Autodesk Fusion 360 part; units mm, degrees
note: some values were not read from the file. Set by a fixed rule: which face or edge a step refers to.
(part 20 of 20)
  spline S58 degree 5 poles (-8.3931, 13.6219) (-8.3929, 13.6198) (-8.3924, 13.6155) (-8.3916, 13.6092) (-8.3906, 13.6008) (-8.3893, 13.5903) (-8.3879, 13.5798) (-8.3866, 13.5693) (-8.3853, 13.5589) (-8.3839, 13.5485) (-8.3826, 13.5382) (-8.3812, 13.5278) (-8.3798, 13.5175) (-8.3784, 13.5072) (-8.377, 13.497) (-8.3755, 13.4867) (-8.3741, 13.4766) (-8.3726, 13.4664) (-8.3712, 13.4563) (-8.3697, 13.4461) (-8.3682, 13.4361) (-8.3667, 13.426) (-8.3652, 13.416) (-8.3637, 13.406) (-8.3621, 13.396) (-8.3606, 13.3861) (-8.359, 13.3762) (-8.3574, 13.3663) (-8.3558, 13.3565) (-8.3542, 13.3467) (-8.3526, 13.3369) (-8.351, 13.3272) (-8.3494, 13.3174) (-8.3477, 13.3078) (-8.3461, 13.2981) (-8.3444, 13.2885) (-8.3427, 13.2789) (-8.341, 13.2693) (-8.3393, 13.2598) (-8.3376, 13.2503) (-8.3359, 13.2408) (-8.3342, 13.2313) (-8.3324, 13.2219) (-8.3307, 13.2125) (-8.3289, 13.2032) (-8.3271, 13.1939) (-8.3254, 13.1846) (-8.3236, 13.1753) (-8.3218, 13.1661) (-8.3199, 13.1569) (-8.3181, 13.1478) (-8.3163, 13.1386) (-8.3145, 13.1296) (-8.3126, 13.1205) (-8.3107, 13.1115) (-8.3089, 13.1025) (-8.307, 13.0935) (-8.3051, 13.0846) (-8.3032, 13.0757) (-8.3013, 13.0668) (-8.2994, 13.058) (-8.2975, 13.0492) (-8.2956, 13.0404) (-8.2936, 13.0317) (-8.2917, 13.023) (-8.2897, 13.0143) (-8.2878, 13.0057) (-8.2858, 12.9971) (-8.2838, 12.9885) (-8.2818, 12.98) (-8.2799, 12.9715) (-8.2779, 12.963) (-8.2759, 12.9546) (-8.2738, 12.9462) (-8.2718, 12.9379) (-8.2698, 12.9295) (-8.2678, 12.9212) (-8.2657, 12.913) (-8.2637, 12.9048) (-8.2616, 12.8966) (-8.2596, 12.8884) (-8.2575, 12.8803) (-8.2554, 12.8722) (-8.2534, 12.8642) (-8.2513, 12.8562) (-8.2492, 12.8482) (-8.2471, 12.8403) (-8.245, 12.8324) (-8.2429, 12.8245) (-8.2408, 12.8167) (-8.2387, 12.8089) (-8.2366, 12.8011) (-8.2345, 12.7934) (-8.2323, 12.7857) (-8.2302, 12.7781) (-8.2281, 12.7705) (-8.2259, 12.7629) (-8.2238, 12.7554) (-8.2216, 12.7479) (-8.2195, 12.7404) (-8.2173, 12.733) (-8.2152, 12.7256) (-8.213, 12.7183) (-8.2109, 12.711) (-8.2087, 12.7037) (-8.2065, 12.6965) (-8.2044, 12.6893) (-8.2022, 12.6821) (-8.2, 12.675) (-8.1978, 12.6679) (-8.1956, 12.6609) (-8.1935, 12.6539) (-8.1913, 12.6469) (-8.1891, 12.64) (-8.1869, 12.6331) (-8.1847, 12.6263) (-8.1825, 12.6195) (-8.1803, 12.6127) (-8.1782, 12.606) (-8.176, 12.5993) (-8.1738, 12.5926) (-8.1716, 12.586) (-8.1694, 12.5795) (-8.1672, 12.5729) (-8.165, 12.5665) (-8.1628, 12.56) (-8.1606, 12.5536) (-8.1584, 12.5473) (-8.1563, 12.5409) (-8.1541, 12.5347) (-8.1519, 12.5284) (-8.1497, 12.5222) (-8.1475, 12.5161) (-8.1453, 12.51) (-8.1432, 12.5039) (-8.141, 12.4979) (-8.1388, 12.4919) (-8.1366, 12.4859) (-8.1345, 12.48) (-8.1323, 12.4742) (-8.1302, 12.4683) (-8.128, 12.4626) (-8.1258, 12.4568) (-8.1237, 12.4512) (-8.1215, 12.4455) (-8.1194, 12.4399) (-8.1173, 12.4344) (-8.1151, 12.4289) (-8.113, 12.4234) (-8.1109, 12.418) (-8.1088, 12.4126) (-8.1067, 12.4073) (-8.1046, 12.402) (-8.1025, 12.3967) (-8.1004, 12.3915) (-8.0983, 12.3864) (-8.0962, 12.3813) (-8.0941, 12.3762) (-8.0921, 12.3712) (-8.09, 12.3662) (-8.088, 12.3613) (-8.0859, 12.3564) (-8.0839, 12.3516) (-8.0819, 12.3468) (-8.0799, 12.3421) (-8.0779, 12.3374) (-8.0759, 12.3327) (-8.0739, 12.3281) (-8.0719, 12.3236) (-8.0699, 12.3191) (-8.068, 12.3146) (-8.066, 12.3102) (-8.0641, 12.3059) (-8.0622, 12.3016) (-8.0603, 12.2973) (-8.0584, 12.2931) (-8.0565, 12.289) (-8.0546, 12.2848) (-8.0527, 12.2808) (-8.0509, 12.2768) (-8.0491, 12.2728) (-8.0472, 12.2689) (-8.0454, 12.265) (-8.0436, 12.2612) (-8.0419, 12.2575) (-8.0401, 12.2538) (-8.0383, 12.2501) (-8.0366, 12.2465) (-8.0349, 12.243) (-8.0332, 12.2395) (-8.0315, 12.236) (-8.0298, 12.2326) (-8.0282, 12.2293) (-8.0265, 12.226) (-8.0249, 12.2228) (-8.0233, 12.2196) (-8.0218, 12.2164) (-8.0202, 12.2134) (-8.0187, 12.2104) (-8.0171, 12.2074) (-8.0156, 12.2045) (-8.0142, 12.2016) (-8.0127, 12.1988) (-8.0113, 12.1961) (-8.0098, 12.1934) (-8.0084, 12.1908) (-8.0071, 12.1882) (-8.0057, 12.1857) (-8.0044, 12.1832) (-8.0031, 12.1808) (-8.0018, 12.1785) (-8.0006, 12.1762) (-7.9994, 12.1739) (-7.9982, 12.1718) (-7.997, 12.1696) (-7.9958, 12.1676) (-7.9947, 12.1656) (-7.9936, 12.1637) (-7.9926, 12.1618) (-7.9915, 12.16) (-7.9905, 12.1582) (-7.9896, 12.1565) (-7.9886, 12.1549) (-7.9877, 12.1533) (-7.9868, 12.1518) (-7.986, 12.1504) (-7.9852, 12.149) (-7.9844, 12.1477) (-7.9836, 12.1464) (-7.9829, 12.1452) (-7.9823, 12.1441) (-7.9816, 12.1431) (-7.981, 12.1421) (-7.9804, 12.1411) (-7.9799, 12.1403) (-7.9794, 12.1395) (-7.979, 12.1388) (-7.9786, 12.1381) (-7.9782, 12.1375) (-7.9779, 12.137) (-7.9776, 12.1365) (-7.9774, 12.1362) (-7.9772, 12.136) (-7.9772, 12.1359) (-7.9771, 12.1359) knots -1 -1 -1 -1 -1 -1 -0.99583333 -0.99166667 -0.9875 -0.98333333 -0.97916667 -0.975 -0.97083333 -0.96666667 -0.9625 -0.95833333 -0.95416667 -0.95 -0.94583333 -0.94166667 -0.9375 -0.93333333 -0.92916667 -0.925 -0.92083333 -0.91666667 -0.9125 -0.90833333 -0.90416667 -0.9 -0.89583333 -0.89166667 -0.8875 -0.88333333 -0.87916667 -0.875 -0.87083333 -0.86666667 -0.8625 -0.85833333 -0.85416667 -0.85 -0.84583333 -0.84166667 -0.8375 -0.83333333 -0.82916667 -0.825 -0.82083333 -0.81666667 -0.8125 -0.80833333 -0.80416667 -0.8 -0.79583333 -0.79166667 -0.7875 -0.78333333 -0.77916667 -0.775 -0.77083333 -0.76666667 -0.7625 -0.75833333 -0.75416667 -0.75 -0.74583333 -0.74166667 -0.7375 -0.73333333 -0.72916667 -0.725 -0.72083333 -0.71666667 -0.7125 -0.70833333 -0.70416667 -0.7 -0.69583333 -0.69166667 -0.6875 -0.68333333 -0.67916667 -0.675 -0.67083333 -0.66666667 -0.6625 -0.65833333 -0.65416667 -0.65 -0.64583333 -0.64166667 -0.6375 -0.63333333 -0.62916667 -0.625 -0.62083333 -0.61666667 -0.6125 -0.60833333 -0.60416667 -0.6 -0.59583333 -0.59166667 -0.5875 -0.58333333 -0.57916667 -0.575 -0.57083333 -0.56666667 -0.5625 -0.55833333 -0.55416667 -0.55 -0.54583333 -0.54166667 -0.5375 -0.53333333 -0.52916667 -0.525 -0.52083333 -0.51666667 -0.5125 -0.50833333 -0.50416667 -0.5 -0.49583333 -0.49166667 -0.4875 -0.48333333 -0.47916667 -0.475 -0.47083333 -0.46666667 -0.4625 -0.45833333 -0.45416667 -0.45 -0.44583333 -0.44166667 -0.4375 -0.43333333 -0.42916667 -0.425 -0.42083333 -0.41666667 -0.4125 -0.40833333 -0.40416667 -0.4 -0.39583333 -0.39166667 -0.3875 -0.38333333 -0.37916667 -0.375 -0.37083333 -0.36666667 -0.3625 -0.35833333 -0.35416667 -0.35 -0.34583333 -0.34166667 -0.3375 -0.33333333 -0.32916667 -0.325 -0.32083333 -0.31666667 -0.3125 -0.30833333 -0.30416667 -0.3 -0.29583333 -0.29166667 -0.2875 -0.28333333 -0.27916667 -0.275 -0.27083333 -0.26666667 -0.2625 -0.25833333 -0.25416667 -0.25 -0.24583333 -0.24166667 -0.2375 -0.23333333 -0.22916667 -0.225 -0.22083333 -0.21666667 -0.2125 -0.20833333 -0.20416667 -0.2 -0.19583333 -0.19166667 -0.1875 -0.18333333 -0.17916667 -0.175 -0.17083333 -0.16666667 -0.1625 -0.15833333 -0.15416667 -0.15 -0.14583333 -0.14166667 -0.1375 -0.13333333 -0.12916667 -0.125 -0.12083333 -0.11666667 -0.1125 -0.10833333 -0.10416667 -0.1 -0.09583333 -0.09166667 -0.0875 -0.08333333 -0.07916667 -0.075 -0.07083333 -0.06666667 -0.0625 -0.05833333 -0.05416667 -0.05 -0.04583333 -0.04166667 -0.0375 -0.03333333 -0.02916667 -0.025 -0.02083333 -0.01666667 -0.0125 -0.00833333 -0.00416667 0 0 0 0 0 0
  line L116 (-7.9771, 12.1359) -> (-7.9768, 12.1353)
  line L117 (-7.9768, 12.1353) -> (-7.5526, 11.49)
  arc A58 (-7.5526, 11.49) -> (-8.5938, 10.7336) centre (0, 0) ccw
  line L118 (-8.5938, 10.7336) -> (-9.0764, 11.3364)
  line L119 (-9.0764, 11.3364) -> (-9.0768, 11.3369)
  spline S59 degree 5 poles (-9.0768, 11.3369) (-9.0769, 11.3369) (-9.0769, 11.337) (-9.0771, 11.3372) (-9.0773, 11.3375) (-9.0777, 11.3379) (-9.0781, 11.3384) (-9.0785, 11.3389) (-9.079, 11.3395) (-9.0796, 11.3402) (-9.0802, 11.3409) (-9.0808, 11.3417) (-9.0815, 11.3425) (-9.0823, 11.3434) (-9.0831, 11.3443) (-9.084, 11.3453) (-9.0849, 11.3464) (-9.0858, 11.3475) (-9.0868, 11.3486) (-9.0879, 11.3498) (-9.089, 11.3511) (-9.0902, 11.3524) (-9.0914, 11.3537) (-9.0926, 11.3551) (-9.0939, 11.3566) (-9.0953, 11.3581) (-9.0967, 11.3596) (-9.0982, 11.3612) (-9.0997, 11.3628) (-9.1012, 11.3645) (-9.1028, 11.3662) (-9.1045, 11.368) (-9.1062, 11.3698) (-9.1079, 11.3717) (-9.1097, 11.3735) (-9.1115, 11.3755) (-9.1134, 11.3775) (-9.1153, 11.3795) (-9.1173, 11.3815) (-9.1194, 11.3836) (-9.1214, 11.3858) (-9.1235, 11.388) (-9.1257, 11.3902) (-9.1279, 11.3924) (-9.1302, 11.3947) (-9.1325, 11.397) (-9.1348, 11.3994) (-9.1372, 11.4018) (-9.1397, 11.4042) (-9.1422, 11.4067) (-9.1447, 11.4092) (-9.1473, 11.4117) (-9.1499, 11.4143) (-9.1526, 11.4169) (-9.1553, 11.4195) (-9.158, 11.4222) (-9.1608, 11.4249) (-9.1637, 11.4276) (-9.1666, 11.4304) (-9.1695, 11.4332) (-9.1725, 11.436) (-9.1755, 11.4389) (-9.1786, 11.4418) (-9.1817, 11.4447) (-9.1848, 11.4476) (-9.188, 11.4506) (-9.1913, 11.4536) (-9.1946, 11.4566) (-9.1979, 11.4597) (-9.2013, 11.4627) (-9.2047, 11.4658) (-9.2081, 11.469) (-9.2116, 11.4721) (-9.2152, 11.4753) (-9.2188, 11.4785) (-9.2224, 11.4818) (-9.2261, 11.485) (-9.2298, 11.4883) (-9.2335, 11.4916) (-9.2373, 11.495) (-9.2412, 11.4983) (-9.2451, 11.5017) (-9.249, 11.5051) (-9.253, 11.5085) (-9.257, 11.512) (-9.261, 11.5154) (-9.2651, 11.5189) (-9.2692, 11.5224) (-9.2734, 11.526) (-9.2776, 11.5295) (-9.2819, 11.5331) (-9.2862, 11.5367) (-9.2905, 11.5403) (-9.2949, 11.544) (-9.2993, 11.5476) (-9.3038, 11.5513) (-9.3083, 11.555) (-9.3128, 11.5587) (-9.3174, 11.5624) (-9.322, 11.5662) (-9.3267, 11.5699) (-9.3314, 11.5737) (-9.3361, 11.5775) (-9.3409, 11.5813) (-9.3457, 11.5852) (-9.3506, 11.589) (-9.3555, 11.5929) (-9.3605, 11.5968) (-9.3654, 11.6007) (-9.3705, 11.6046) (-9.3755, 11.6085) (-9.3806, 11.6125) (-9.3858, 11.6164) (-9.3909, 11.6204) (-9.3962, 11.6244) (-9.4014, 11.6284) (-9.4067, 11.6324) (-9.412, 11.6365) (-9.4174, 11.6405) (-9.4228, 11.6446) (-9.4283, 11.6486) (-9.4338, 11.6527) (-9.4393, 11.6568) (-9.4449, 11.6609) (-9.4505, 11.6651) (-9.4561, 11.6692) (-9.4618, 11.6733) (-9.4675, 11.6775) (-9.4733, 11.6817) (-9.4791, 11.6859) (-9.4849, 11.6901) (-9.4908, 11.6943) (-9.4967, 11.6985) (-9.5026, 11.7027) (-9.5086, 11.707) (-9.5146, 11.7112) (-9.5207, 11.7155) (-9.5268, 11.7197) (-9.5329, 11.724) (-9.5391, 11.7283) (-9.5453, 11.7326) (-9.5516, 11.7369) (-9.5578, 11.7412) (-9.5642, 11.7455) (-9.5705, 11.7499) (-9.5769, 11.7542) (-9.5833, 11.7586) (-9.5898, 11.7629) (-9.5963, 11.7673) (-9.6028, 11.7717) (-9.6094, 11.776) (-9.616, 11.7804) (-9.6227, 11.7848) (-9.6294, 11.7892) (-9.6361, 11.7936) (-9.6428, 11.798) (-9.6496, 11.8025) (-9.6565, 11.8069) (-9.6633, 11.8113) (-9.6702, 11.8158) (-9.6772, 11.8202) (-9.6841, 11.8247) (-9.6912, 11.8291) (-9.6982, 11.8336) (-9.7053, 11.8381) (-9.7124, 11.8425) (-9.7195, 11.847) (-9.7267, 11.8515) (-9.7339, 11.856) (-9.7412, 11.8605) (-9.7485, 11.865) (-9.7558, 11.8695) (-9.7632, 11.874) (-9.7706, 11.8785) (-9.778, 11.883) (-9.7855, 11.8875) (-9.793, 11.8921) (-9.8005, 11.8966) (-9.8081, 11.9011) (-9.8157, 11.9056) (-9.8233, 11.9102) (-9.831, 11.9147) (-9.8387, 11.9193) (-9.8464, 11.9238) (-9.8542, 11.9283) (-9.862, 11.9329) (-9.8699, 11.9374) (-9.8777, 11.942) (-9.8857, 11.9465) (-9.8936, 11.9511) (-9.9016, 11.9557) (-9.9096, 11.9602) (-9.9176, 11.9648) (-9.9257, 11.9693) (-9.9338, 11.9739) (-9.942, 11.9785) (-9.9502, 11.983) (-9.9584, 11.9876) (-9.9666, 11.9921) (-9.9749, 11.9967) (-9.9832, 12.0013) (-9.9916, 12.0058) (-9.9999, 12.0104) (-10.0084, 12.015) (-10.0168, 12.0195) (-10.0253, 12.0241) (-10.0338, 12.0287) (-10.0423, 12.0332) (-10.0509, 12.0378) (-10.0595, 12.0423) (-10.0682, 12.0469) (-10.0768, 12.0515) (-10.0855, 12.056) (-10.0943, 12.0606) (-10.1031, 12.0651) (-10.1119, 12.0697) (-10.1207, 12.0743) (-10.1296, 12.0788) (-10.1385, 12.0834) (-10.1474, 12.0879) (-10.1564, 12.0924) (-10.1654, 12.097) (-10.1744, 12.1015) (-10.1834, 12.1061) (-10.1925, 12.1106) (-10.2017, 12.1151) (-10.2108, 12.1197) (-10.22, 12.1242) (-10.2292, 12.1287) (-10.2385, 12.1332) (-10.2478, 12.1378) (-10.2571, 12.1423) (-10.2664, 12.1468) (-10.2758, 12.1513) (-10.2852, 12.1558) (-10.2946, 12.1603) (-10.3041, 12.1648) (-10.3136, 12.1693) (-10.3231, 12.1738) (-10.3327, 12.1783) (-10.3423, 12.1828) (-10.35, 12.1863) (-10.3558, 12.189) (-10.3596, 12.1908) (-10.3616, 12.1917) knots 0 0 0 0 0 0 0.00416667 0.00833333 0.0125 0.01666667 0.02083333 0.025 0.02916667 0.03333333 0.0375 0.04166667 0.04583333 0.05 0.05416667 0.05833333 0.0625 0.06666667 0.07083333 0.075 0.07916667 0.08333333 0.0875 0.09166667 0.09583333 0.1 0.10416667 0.10833333 0.1125 0.11666667 0.12083333 0.125 0.12916667 0.13333333 0.1375 0.14166667 0.14583333 0.15 0.15416667 0.15833333 0.1625 0.16666667 0.17083333 0.175 0.17916667 0.18333333 0.1875 0.19166667 0.19583333 0.2 0.20416667 0.20833333 0.2125 0.21666667 0.22083333 0.225 0.22916667 0.23333333 0.2375 0.24166667 0.24583333 0.25 0.25416667 0.25833333 0.2625 0.26666667 0.27083333 0.275 0.27916667 0.28333333 0.2875 0.29166667 0.29583333 0.3 0.30416667 0.30833333 0.3125 0.31666667 0.32083333 0.325 0.32916667 0.33333333 0.3375 0.34166667 0.34583333 0.35 0.35416667 0.35833333 0.3625 0.36666667 0.37083333 0.375 0.37916667 0.38333333 0.3875 0.39166667 0.39583333 0.4 0.40416667 0.40833333 0.4125 0.41666667 0.42083333 0.425 0.42916667 0.43333333 0.4375 0.44166667 0.44583333 0.45 0.45416667 0.45833333 0.4625 0.46666667 0.47083333 0.475 0.47916667 0.48333333 0.4875 0.49166667 0.49583333 0.5 0.50416667 0.50833333 0.5125 0.51666667 0.52083333 0.525 0.52916667 0.53333333 0.5375 0.54166667 0.54583333 0.55 0.55416667 0.55833333 0.5625 0.56666667 0.57083333 0.575 0.57916667 0.58333333 0.5875 0.59166667 0.59583333 0.6 0.60416667 0.60833333 0.6125 0.61666667 0.62083333 0.625 0.62916667 0.63333333 0.6375 0.64166667 0.64583333 0.65 0.65416667 0.65833333 0.6625 0.66666667 0.67083333 0.675 0.67916667 0.68333333 0.6875 0.69166667 0.69583333 0.7 0.70416667 0.70833333 0.7125 0.71666667 0.72083333 0.725 0.72916667 0.73333333 0.7375 0.74166667 0.74583333 0.75 0.75416667 0.75833333 0.7625 0.76666667 0.77083333 0.775 0.77916667 0.78333333 0.7875 0.79166667 0.79583333 0.8 0.80416667 0.80833333 0.8125 0.81666667 0.82083333 0.825 0.82916667 0.83333333 0.8375 0.84166667 0.84583333 0.85 0.85416667 0.85833333 0.8625 0.86666667 0.87083333 0.875 0.87916667 0.88333333 0.8875 0.89166667 0.89583333 0.9 0.90416667 0.90833333 0.9125 0.91666667 0.92083333 0.925 0.92916667 0.93333333 0.9375 0.94166667 0.94583333 0.95 0.95416667 0.95833333 0.9625 0.96666667 0.97083333 0.975 0.97916667 0.98333333 0.9875 0.99166667 0.99583333 1 1 1 1 1 1
  arc A59 (-10.3616, 12.1917) -> (-11.0419, 11.5792) centre (0, 0) ccw
  arc A60 (-0.3, 3) -> (-0.3, -3) centre (-0.3, 0) ccw
  line L120 (-0.3, 3) -> (-0.3, -3)
  line L121 (0.3, -3) -> (0.3, 3)
  arc A61 (0.3, -3) -> (0.3, 3) centre (0.3, 0) ccw
  circle A62 centre (10, 0) radius 1.7
  circle A63 centre (0, 10) radius 1.7
  circle A64 centre (0, -10) radius 1.7
  circle A65 centre (-10, 0) radius 1.7
  circle A66 centre (-7.0711, -7.0711) radius 1.7
  circle A67 centre (-7.0711, 7.0711) radius 1.7
  circle A68 centre (7.0711, -7.0711) radius 1.7
  circle A69 centre (7.0711, 7.0711) radius 1.7
  circle A70 centre (0, 0) radius 13.5
  dimension "d24" = 27
  constraint concentric A0 A70
  measures "d24" diameter of A70
extrude "押し出し5" cut sketch "スケッチ6" against normal blind 3 contours S0 L1 A0 L2 S1 A1 S2 L5 A2 L6 S3 A3 S4 L9 A4 L10 S5 A5 S6 L13 A6 L14 S7 A7 S8 L17 A8 L18 S9 A9 S10 L21 A10 L22 S11 A11 S12 L25 A12 L26 S13 A13 S14 L29 A14 L30 S15 A15 S16 L33 A16 L34 S17 A17 S18 L37 A18 L38 S19 A19 S20 L41 A20 L42 S21 A21 S22 L45 A22 L46 S23 A23 S24 L49 A24 L50 S25 A25 S26 L53 A26 L54 S27 A27 S28 L57 A28 L58 S29 A29 S30 L61 A30 L62 S31 A31 S32 L65 A32 L66 S33 A33 S34 L69 A34 L70 S35 A35 S36 L73 A36 L74 S37 A37 S38 L77 A38 L78 S39 A39 S40 L81 A40 L82 S41 A41 S42 L85 A42 L86 S43 A43 S44 L89 A44 L90 S45 A45 S46 L93 A46 L94 S47 A47 S48 L97 A48 L98 S49 A49 S50 L101 A50 L102 S51 A51 S52 L105 A52 L106 S53 A53 S54 L109 A54 L110 S55 A55 S56 L113 A56 L114 S57 A57 S58 L117 A58 L118 S59 A59
extrude "押し出し6" add 1 faces at (2.4936, 5.9882, 3) along direction (0, 0, 1) blind 5
delete_face "面を削除1" 2 faces at (0.3, -1, 6.3333) (0.3, 1, 2)
delete_face "面を削除2" 2 faces at (-2.2284, 2.2981, 6.3333) (-2.1114, -2.3914, 1)
sketch "スケッチ7" plane through (0, 0, 8) normal (0, 0, 1) x (-1, 0, 0)
  circle A0 centre (0, 0) radius 13.5
  circle A1 centre (10, 0) radius 1.7
  circle A2 centre (0, 10) radius 1.7
  circle A3 centre (0, -10) radius 1.7
  circle A4 centre (-10, 0) radius 1.7
  circle A5 centre (-7.0711, -7.0711) radius 1.7
  circle A6 centre (-7.0711, 7.0711) radius 1.7
  circle A7 centre (7.0711, -7.0711) radius 1.7
  circle A8 centre (7.0711, 7.0711) radius 1.7
  circle A9 centre (0, -10) radius 2.1
  circle A10 centre (7.0711, -7.0711) radius 2.1
  circle A11 centre (10, 0) radius 2.1
  circle A12 centre (7.0711, 7.0711) radius 2.1
  circle A13 centre (0, 10) radius 2.1
  circle A14 centre (-7.0711, 7.0711) radius 2.1
  circle A15 centre (-10, 0) radius 2.1
  circle A16 centre (-7.0711, -7.0711) radius 2.1
  dimension "d29" = 4.2
  dimension "d31" = 360
  constraint concentric A3 A9
  measures "d29" diameter of A9
extrude "押し出し7" cut sketch "スケッチ7" against normal blind 8 contours A9 | A10 | A11 | A12 | A13 | A14 | A15 | A16
